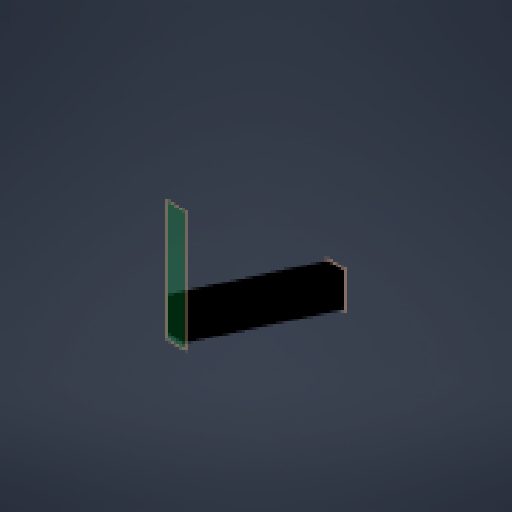
# Autodesk Inventor part: UpperNoseDiagonalsv2
Saved by Autodesk Inventor 2027 (Build 310192000, 192)
## iProperties
Created: 2026-08-07
Part Number: UpperNoseDiagonalsv2
Material: Generic
Document SubType Name: Modeling
Designer: lucas
Density: 1 g/cm^3
Appearance: Default
Author: lucas
Autodesk Inventor part; units mm, degrees
ref_plane "YZ Plane" through (0, 0, 0) normal (1, 0, 0) x (0, 1, 0)
ref_plane "XZ Plane" through (0, 0, 0) normal (0, 1, 0) x (-1, 0, 0)
ref_plane "XY Plane" through (0, 0, 0) normal (0, 0, 1) x (1, 0, 0)
ref_plane "Work Plane1" through (0, 0, 0) normal (0, 0, 1) x (1, 0, 0)
sketch "Sketch1" plane through (0, 0, 0) normal (0, 0, 1) x (1, 0, 0)
  line L0 (0, 0) -> (0, 101.6) projected
  line L1 (0, 101.6) -> (-50.8, 101.6) projected
  line L2 (-50.8, 0) -> (-50.8, 101.6) projected
  line L3 (0, 0) -> (-50.8, 0) projected
  line L4 (-50.8, 0) -> (0, 0)
  line L5 (0, 0) -> (0, 101.6)
  line L6 (0, 101.6) -> (-50.8, 101.6)
  line L7 (-50.8, 101.6) -> (-50.8, 0)
  constraints: 8 end point, 2 parallel, 1 horizontal, 1 perpendicular
ref_plane "Work Plane2" through (177.8, 711.2, 711.4062) normal (0, 0, -1) x (1, 0, 0)
sketch "Sketch2" plane through (177.8, 711.2, 711.4062) normal (0, 0, -1) x (1, 0, 0)
  line L0 (0, 330.2) -> (50.8, 330.2)
  line L1 (50.8, 330.2) -> (50.8, 228.6)
  line L2 (50.8, 228.6) -> (0, 228.6)
  line L3 (0, 228.6) -> (0, 330.2)
  point P0 (-177.8, 711.2)
  dimension "d0" = 50.8
  dimension "d1" = 101.6
  constraints: 8 end point, 2 parallel, 1 horizontal, 1 perpendicular, 1 other
  measures "d0" distance of L0.start L0.end
  measures "d1" distance of L0.end L1.end
loft "Loft1" add profiles "Sketch1", "Sketch2"
body "Solid1"
